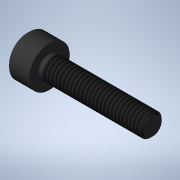
# Autodesk Inventor part: BOLT3-14
Saved by Autodesk Inventor 2021 (Build 250183000, 183)
## iProperties
Created: 2025-09-06
Part Number: BOLT3-14
Material: Generic
Catalog Web Link: www.cadenas.de
Description: BOLT-Hexagon Socket Head Cap Screws
Vendor: MISUMI
Document SubType Name: Modeling
Designer: psAdmin
Manufacturer: MISUMI
Mass: 0.160406 g
Surface Area: 2.39495 cm^2
Volume: 0.160406 cm^3
Density: 1 g/cm^3
Appearance: PSOLRGB-175-175-175
Category: PARTsolutions
Company: MISUMI
Title: BOLT3-14
Author: Cadenas PARTsolutions
Comments: Hexagon Socket Head Cap Screws
PSOL_IDENT_0: {$CADENAS_DATA/23d-libs/misumi/metric/accessories/bolt.prj},156 {VTYP=3D},{NB=BOLT3-14},{LINA=BOLT3-
PSOL_IDENT_1: 14},{NN=BOLT},{DATE=29.11.2024 04:47:06},{GEOMDATE=12.05.2017 08:21:09},{VERSION=},{LINEID=60},{WBVA
PSOL_IDENT_2: R=L},{WBNUMERIC=L}  {NB=BOLT3-14},{LINA=BOLT3-14},{KT=DUMMY},{PN=BOLT3-14},{TYPE=BOLT},{L=14.0},{M=3
PSOL_IDENT_3: .0},{P=0.5},{A=5.5},{E=3.0},{B=2.5},{C=0.30},{LL=0}
NB: BOLT3-14
NN: BOLT
NT: Hexagon Socket Head Cap Screws
NBSYN: $PN.
LINA: BOLT3-14
CATALOG: Misumi
PN: BOLT3-14
L: 14
M: 3
P: 0.5
C: 0.3
SUPPLIER: MISUMI
ARTICLENO: BOLT3-14
BOMINFO: BOLT3-14
CREATOR: CADENAS GmbH
Autodesk Inventor part; units mm, degrees
sketch "Sketch_1" plane through (0, 0, 0) normal (0, 0, 1) x (1, 0, 0)
  line L0 (14, 0) -> (-3, 0)
  line L1 (-3, 0) -> (-3, 2.45)
  line L2 (-3, 2.45) -> (-2.7, 2.75)
  line L3 (-2.7, 2.75) -> (0, 2.75)
  line L4 (0, 2.75) -> (0, 1.5)
  line L5 (0, 1.5) -> (13.6935, 1.5)
  line L6 (13.6935, 1.5) -> (14, 1.1935)
  line L7 (14, 1.1935) -> (14, 0)
  line L8 (14, 0) -> (-3, 0)
  constraints: 18 end point
revolve "Revolution1" add sketch "Sketch_1" angle 360 about axis through (14, 0, 0) along (1, 0, 0)
thread "Thread1" size "M3x0.5" class "6g" standard "ISO Metric profile" length 13.5 offset 0.5
sketch "Sketch2" plane through (-3, 0, 0) normal (-1, 0, 0) x (0, 0, 1)
  point P0 (0, 0)
hole "Hole1" at (-3, 0, 0) direction (1, 0, 0) diameter 2.5 depth 1.5 tip angle 150
sketch "Sketch_3" plane through (-3, 0, 0) normal (1, 0, 0) x (0, 0, -1)
  line L0 (-1.25, -0.7217) -> (0, -1.4434)
  line L1 (0, -1.4434) -> (1.25, -0.7217)
  line L2 (1.25, -0.7217) -> (1.25, 0.7217)
  line L3 (1.25, 0.7217) -> (0, 1.4434)
  line L4 (0, 1.4434) -> (-1.25, 0.7217)
  line L5 (-1.25, 0.7217) -> (-1.25, -0.7217)
  constraints: 12 end point
extrude "Extrusion1" cut sketch "Sketch_3" along normal blind 1.5
ref_plane "to_cp_XY" through (0, 0, 0) normal (1, 0, 0) x (0, 0, -1)
ref_plane "to_cp_YZ" through (0, 0, 0) normal (0, 0, -1) x (0, 1, 0)
ref_plane "to_cp_ZX" through (0, 0, 0) normal (0, 1, 0) x (1, 0, 0)
body "Solid1"
